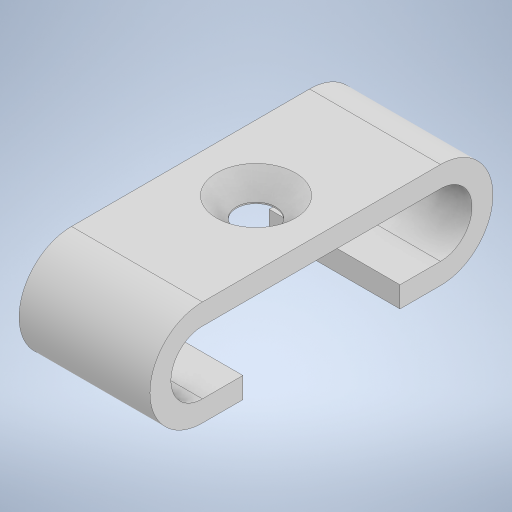
# Autodesk Inventor part: klips
Saved by Autodesk Inventor 2023.4 (Build 274418000, 418)
## iProperties
Created: 2024-08-08
Part Number: klips
Material: Generic
Document SubType Name: Modeling
Designer: komputer
Density: 1 g/cm^3
Appearance: Default
Author: komputer
Autodesk Inventor part; units mm, degrees
ref_plane "YZ Plane" through (0, 0, 0) normal (1, 0, 0) x (0, 1, 0)
ref_plane "XZ Plane" through (0, 0, 0) normal (0, 1, 0) x (-1, 0, 0)
ref_plane "XY Plane" through (0, 0, 0) normal (0, 0, 1) x (1, 0, 0)
sketch "Sketch1" plane through (0, 0, 0) normal (1, 0, 0) x (0, 1, 0)
  line L0 (-5.4603, 8.273) -> (-5.4603, 11.3688)
  line L1 (-0.652, 11.3688) -> (-0.652, 8.273)
  arc A0 (-0.652, 11.3688) -> (-5.4603, 11.3688) centre (-3.0561, 11.3688) ccw
  line L2 (0.948, 8.273) -> (0.948, 11.3688)
  arc A1 (0.948, 11.3688) -> (-7.0603, 11.3688) centre (-3.0561, 11.3688) ccw
  line L3 (-7.0603, 11.3688) -> (-7.0603, 8.273)
  line L4 (-7.0603, 8.273) -> (-5.4603, 8.273)
  line L5 (-0.652, 8.273) -> (-0.652, -3.727)
  line L6 (-3.0561, 13.773) -> (-3.0561, 8.273)
  line L7 (0.948, 8.273) -> (0.948, -3.727)
  line L8 (-0.652, 2.273) -> (-9.3077, 2.273)
  line L9 (-5.4603, -3.727) -> (-5.4603, -6.8229)
  line L10 (-0.652, -6.8229) -> (-0.652, -3.727)
  arc A2 (-5.4603, -6.8229) -> (-0.652, -6.8229) centre (-3.0561, -6.8229) ccw
  line L11 (0.948, -3.727) -> (0.948, -6.8229)
  arc A3 (-7.0603, -6.8229) -> (0.948, -6.8229) centre (-3.0561, -6.8229) ccw
  line L12 (-7.0603, -6.8229) -> (-7.0603, -3.727)
  line L13 (0.948, -3.727) -> (0.948, 8.273)
  line L14 (-7.0603, -3.727) -> (-5.4603, -3.727)
  point P0 (0, 0)
  dimension "d3" = 1.6
  dimension "d4" = 12
  dimension "d5" = 5.5
  constraints: 30 end point, 9 point on circle, 9 symmetric about line, 5 vertical, 4 centre point, 3 horizontal, 3 horizontal alignment, 2 tangent, 1 midpoint, 4 other
  measures "d3" distance between parallel lines of L1 L2
  measures "d4" distance of L1.end L5.end
  measures "d5" distance of L6.start L6.end
extrude "Extrusion1" add sketch "Sketch1" along normal blind 10
sketch "Sketch2" plane through (0, 0.948, 11.3688) normal (0, 1, 0) x (1, 0, 0)
  line L0 (0, 18.1917) -> (0, 0) projected
  line L1 (0, 0) -> (10, 0) projected
  line L2 (10, 18.1917) -> (10, 0) projected
  line L3 (0, 18.1917) -> (10, 18.1917) projected
  point P0 (0, 11.3688)
  point P1 (5, 9.0958)
hole "Hole1" at (5, 0.948, 2.273) direction (0, -1, 0) diameter 3 end through all countersink diameter 6 countersink angle 90
body "Solid1"
